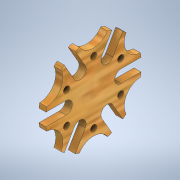
# Autodesk Inventor part: GenevaGear
Saved by Autodesk Inventor 2020.2 (Build 242310000, 310)
## iProperties
Created: 2019-12-15
Part Number: GenevaGear
Material: Plywood, Finish
Document SubType Name: Modeling
Designer: Paul Lefeuvre
Density: 0.552 g/cm^3
Appearance: Plywood - New
Author: Paul Lefeuvre
Autodesk Inventor part; units mm, degrees
ref_plane "YZ Plane" through (0, 0, 0) normal (1, 0, 0) x (0, 1, 0)
ref_plane "XZ Plane" through (0, 0, 0) normal (0, 1, 0) x (-1, 0, 0)
ref_plane "XY Plane" through (0, 0, 0) normal (0, 0, 1) x (1, 0, 0)
sketch "Sketch1" plane through (0, 0, 0) normal (1, 0, 0) x (0, 1, 0)
  circle A0 centre (0, 0) radius 100 construction
  circle A1 centre (0, 0) radius 72.5 construction
  circle A2 centre (0, 0) radius 110 construction
  circle A3 centre (0, 0) radius 61.3705
  line L0 (7.5, -35.1667) -> (7.5, -60.9105) construction
  line L1 (-7.5, -35.1667) -> (-7.5, -60.9105) construction
  arc A4 (7.5, -35.1667) -> (-7.5, -35.1667) centre (0, -35.1667) ccw construction
  line L2 (0, 0) -> (0, -136.3111) construction
  line L3 (8.1, -60.8336) -> (8.1, -35.1667)
  arc A5 (8.1, -35.1667) -> (-8.1, -35.1667) centre (0, -35.1667) ccw
  line L4 (-8.1, -35.1667) -> (-8.1, -60.8336)
  line L5 (56.7334, -23.402) -> (34.5052, -10.5685)
  arc A6 (34.5052, -10.5685) -> (26.4052, -24.5981) centre (30.4552, -17.5833) ccw
  line L6 (26.4052, -24.5981) -> (48.6334, -37.4316)
  line L7 (48.6334, 37.4316) -> (26.4052, 24.5981)
  arc A7 (26.4052, 24.5981) -> (34.5052, 10.5685) centre (30.4552, 17.5833) ccw
  line L8 (34.5052, 10.5685) -> (56.7334, 23.402)
  line L9 (-8.1, 60.8336) -> (-8.1, 35.1667)
  arc A8 (-8.1, 35.1667) -> (8.1, 35.1667) centre (0, 35.1667) ccw
  line L10 (8.1, 35.1667) -> (8.1, 60.8336)
  line L11 (-56.7334, 23.402) -> (-34.5052, 10.5685)
  arc A9 (-34.5052, 10.5685) -> (-26.4052, 24.5981) centre (-30.4552, 17.5833) ccw
  line L12 (-26.4052, 24.5981) -> (-48.6334, 37.4316)
  line L13 (-48.6334, -37.4316) -> (-26.4052, -24.5981)
  arc A10 (-26.4052, -24.5981) -> (-34.5052, -10.5685) centre (-30.4552, -17.5833) ccw
  line L14 (-34.5052, -10.5685) -> (-56.7334, -23.402)
  line L15 (34.2052, -11.0881) -> (56.5, -23.96) construction
  arc A11 (34.2052, -11.0881) -> (26.7052, -24.0785) centre (30.4552, -17.5833) ccw construction
  line L16 (26.7052, -24.0785) -> (49, -36.9504) construction
  circle A12 centre (35.1667, -60.9105) radius 42.6667 construction
  circle A13 centre (35.1667, -60.9105) radius 27.6667 construction
  circle A14 centre (0, 0) radius 27.6667 construction
  line L17 (55, -95.2628) -> (56.5, -97.8609)
  arc A15 (45.0316, -41.6952) -> (13.5933, -59.8461) centre (35.1667, -60.9105) ccw
  arc A16 (58.6249, 18.1509) -> (58.6249, -18.1509) centre (70.3333, 0) ccw
  arc A17 (13.5933, 59.8461) -> (45.0316, 41.6952) centre (35.1667, 60.9105) ccw
  arc A18 (-45.0316, 41.6952) -> (-13.5933, 59.8461) centre (-35.1667, 60.9105) ccw
  arc A19 (-58.6249, -18.1509) -> (-58.6249, 18.1509) centre (-70.3333, 0) ccw
  arc A20 (-13.5933, -59.8461) -> (-45.0316, -41.6952) centre (-35.1667, -60.9105) ccw
  line L18 (0, 0) -> (144.5472, 0) construction
  circle A21 centre (40, 0) radius 3.9
  circle A22 centre (20, 34.641) radius 3.9
  circle A23 centre (-20, 34.641) radius 3.9
  circle A24 centre (-40, 0) radius 3.9
  circle A25 centre (-20, -34.641) radius 3.9
  circle A26 centre (20, -34.641) radius 3.9
  point P0 (-56.7334, 23.402)
  point P1 (-58.6249, 18.1509)
  point P2 (-56.7334, -23.402)
  point P3 (-48.6334, -37.4316)
  point P4 (-45.0316, -41.6952)
  point P5 (-13.5933, -59.8461)
  point P6 (48.6334, -37.4316)
  point P7 (56.7334, -23.402)
  point P8 (58.6249, -18.1509)
  point P9 (58.6249, 18.1509)
  point P10 (56.7334, 23.402)
  point P11 (48.6334, 37.4316)
  point P12 (45.0316, 41.6952)
  point P13 (13.5933, 59.8461)
  point P14 (8.1, 60.8336)
  point P15 (-8.1, 60.8336)
  point P16 (-13.5933, 59.8461)
  point P17 (-45.0316, 41.6952)
  point P18 (-48.6334, 37.4316)
  dimension "d2" = 220
  dimension "d0" = 200
  dimension "d1" = 145
  dimension "d3" = 7.5
  dimension "d4" = 0.6
  dimension "d7" = 360
  dimension "d11" = 60
  dimension "d13" = 15
  dimension "d14" = 3
  dimension "d18" = 360
  dimension "d22" = 7.8
  dimension "d23" = 40
  dimension "d26" = 360
  constraints: 38 end point, 30 point on circle, 25 centre point, 6 tangent, 5 coincident, 3 vertical, 1 horizontal, 1 line through centre, 1 parallel, 1 point on line, 110 other
  measures "d0" diameter of A0
  measures "d1" diameter of A1
  measures "d3" distance between parallel lines of L0 L2
  measures "d4" distance between parallel lines of L0 L3
  measures "d13" radial gap between concentric circles of A12 A13
  measures "d14" distance of L17.start L17.end
  measures "d22" diameter of A21
  measures "d23" distance of A21.centre point (0, 0)
extrude "Extrusion1" add sketch "Sketch1" along normal blind 9 contours A16 A3 L5 A6 L6 A15 L3 A5 L4 A20 L13 A10 L14 A19 L11 A9 L12 A18 L9 A8 L10 A17 L7 A7 L8
body "Solid1"
